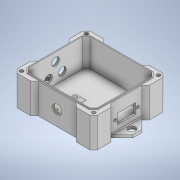
# Autodesk Inventor part: Case
Saved by Autodesk Inventor 2020 (Build 240168000, 168)
## iProperties
Created: 2020-03-10
Part Number: Case
Material: Generic
Document SubType Name: Modeling
Designer: Alex
Density: 1 g/cm^3
Appearance: Default
Author: Alex
Autodesk Inventor part; units mm, degrees
ref_plane "YZ Plane" through (0, 0, 0) normal (1, 0, 0) x (0, 1, 0)
ref_plane "XZ Plane" through (0, 0, 0) normal (0, 1, 0) x (-1, 0, 0)
ref_plane "XY Plane" through (0, 0, 0) normal (0, 0, 1) x (1, 0, 0)
sketch "Sketch1" plane through (0, 0, 0) normal (0, 1, 0) x (-1, 0, 0)
  line L0 (40, -36) -> (-40, -36) construction
  line L1 (-40, -36) -> (-40, 36) construction
  line L2 (-40, 36) -> (40, 36) construction
  line L3 (40, 36) -> (40, -36) construction
  line L4 (21, -36) -> (25, -40)
  line L5 (25, -40) -> (40, -40)
  line L6 (40, -40) -> (44, -36)
  line L7 (44, -36) -> (44, -21)
  line L8 (44, -21) -> (40, -17)
  line L9 (40, 17) -> (44, 21)
  line L10 (44, 21) -> (44, 36)
  line L11 (44, 36) -> (40, 40)
  line L12 (40, 40) -> (25, 40)
  line L13 (25, 40) -> (21, 36)
  line L14 (40, -17) -> (40, 17)
  line L15 (21, -36) -> (-21, -36)
  line L16 (-21, -36) -> (-25, -40)
  line L17 (-25, -40) -> (-40, -40)
  line L18 (-40, -40) -> (-44, -36)
  line L19 (-44, -36) -> (-44, -21)
  line L20 (-44, -21) -> (-40, -17)
  line L21 (-40, -17) -> (-40, 17)
  line L22 (-40, 17) -> (-44, 21)
  line L23 (-44, 21) -> (-44, 36)
  line L24 (-44, 36) -> (-40, 40)
  line L25 (-40, 40) -> (-25, 40)
  line L26 (-25, 40) -> (-21, 36)
  line L27 (21, 36) -> (-21, 36)
  line L28 (40, -36) -> (-40, 36) construction
  line L29 (-40, -36) -> (40, 36) construction
  point P0 (0, 0)
  point P1 (40, 0)
  point P2 (0, -36)
  point P3 (0, 0)
  point P4 (0, 36)
  point P5 (-40, 0)
  dimension "d0" = 4
  dimension "d1" = 80
  dimension "d2" = 72
  dimension "d3" = 4
  dimension "d4" = 4
  dimension "d5" = 4
  dimension "d6" = 135
  dimension "d7" = 0
  dimension "d8" = 15
  constraints: 60 end point, 13 parallel, 10 point on line, 7 equal length, 7 midpoint, 7 perpendicular, 6 collinear, 2 horizontal, 1 coincident, 1 horizontal alignment, 1 vertical alignment
  measures "d0" distance between parallel lines of L5 L0
  measures "d1" distance between parallel lines of L1 L3
  measures "d2" distance of L2.end L0.start
  measures "d3" distance between parallel lines of L7 L3
  measures "d4" distance between parallel lines of L19 L1
  measures "d5" distance between parallel lines of L25 L2
  measures "d6" angle of L15 L16
  measures "d7" distance from line of L17.end L1
  measures "d8" distance of L16.end L17.end
extrude "Extrusion1" add sketch "Sketch1" along normal blind 3
sketch "Sketch2" plane through (0, 3, 0) normal (0, 1, 0) x (1, 0, 0)
  line L0 (21, 36) -> (-21, 36) projected
  line L1 (-21, 36) -> (-25, 40) projected
  line L2 (-25, 40) -> (-40, 40) projected
  line L3 (-40, 40) -> (-44, 36) projected
  line L4 (-44, 36) -> (-44, 21) projected
  line L5 (-44, 21) -> (-40, 17) projected
  line L6 (-40, 17) -> (-40, -17) projected
  line L7 (-40, -17) -> (-44, -21) projected
  line L8 (-44, -21) -> (-44, -36) projected
  line L9 (-44, -36) -> (-40, -40) projected
  line L10 (-40, -40) -> (-25, -40) projected
  line L11 (-25, -40) -> (-21, -36) projected
  line L12 (-21, -36) -> (21, -36) projected
  line L13 (21, -36) -> (25, -40) projected
  line L14 (25, -40) -> (40, -40) projected
  line L15 (40, -40) -> (44, -36) projected
  line L16 (44, -36) -> (44, -21) projected
  line L17 (44, -21) -> (40, -17) projected
  line L18 (40, -17) -> (40, 17) projected
  line L19 (40, 17) -> (44, 21) projected
  line L20 (44, 21) -> (44, 36) projected
  line L21 (44, 36) -> (40, 40) projected
  line L22 (40, 40) -> (25, 40) projected
  line L23 (25, 40) -> (21, 36) projected
  line L24 (-21.8284, 34) -> (21.8284, 34)
  line L25 (21.8284, 34) -> (25.8284, 38) construction
  line L26 (25.8284, 38) -> (39.1716, 38) construction
  line L27 (39.1716, 38) -> (42, 35.1716) construction
  line L28 (42, 35.1716) -> (42, 21.8284) construction
  line L29 (42, 21.8284) -> (38, 17.8284) construction
  line L30 (38, 17.8284) -> (38, -17.8284)
  line L31 (38, -17.8284) -> (42, -21.8284) construction
  line L32 (42, -21.8284) -> (42, -35.1716) construction
  line L33 (42, -35.1716) -> (39.1716, -38) construction
  line L34 (39.1716, -38) -> (25.8284, -38) construction
  line L35 (25.8284, -38) -> (21.8284, -34) construction
  line L36 (21.8284, -34) -> (-21.8284, -34)
  line L37 (-21.8284, -34) -> (-25.8284, -38) construction
  line L38 (-25.8284, -38) -> (-39.1716, -38) construction
  line L39 (-39.1716, -38) -> (-42, -35.1716) construction
  line L40 (-42, -35.1716) -> (-42, -21.8284) construction
  line L41 (-42, -21.8284) -> (-38, -17.8284) construction
  line L42 (-38, -17.8284) -> (-38, 17.8284)
  line L43 (-38, 17.8284) -> (-42, 21.8284) construction
  line L44 (-42, 21.8284) -> (-42, 35.1716) construction
  line L45 (-42, 35.1716) -> (-39.1716, 38) construction
  line L46 (-39.1716, 38) -> (-25.8284, 38) construction
  line L47 (-25.8284, 38) -> (-21.8284, 34) construction
  line L48 (-38, 17.8284) -> (-38, 30)
  line L49 (-38, 30) -> (-34, 34)
  line L50 (-34, 34) -> (-21.8284, 34)
  line L51 (21.8284, 34) -> (34, 34)
  line L52 (34, 34) -> (38, 30)
  line L53 (38, 30) -> (38, 17.8284)
  line L54 (38, -17.8284) -> (38, -30)
  line L55 (38, -30) -> (34, -34)
  line L56 (34, -34) -> (21.8284, -34)
  line L57 (-21.8284, -34) -> (-34, -34)
  line L58 (-34, -34) -> (-38, -30)
  line L59 (-38, -30) -> (-38, -17.8284)
  point P0 (0, 0)
  dimension "d11" = 2
  dimension "d13" = 4
  constraints: 72 end point, 3 equal length, 3 perpendicular, 3 vertical, 2 parallel, 2 point on line, 1 collinear, 1 horizontal, 23 other
  measures "d11" distance between parallel lines of L0 L24
  measures "d13" horizontal distance of L49.end L48.end
extrude "Extrusion2" add sketch "Sketch2" along normal blind 30
sketch "Sketch3" plane through (0, 3, 0) normal (0, 1, 0) x (1, 0, 0)
  line L0 (-34, 34) -> (-38, 30) construction
  line L1 (-38, 30) -> (-38, -30) construction
  line L2 (-38, -30) -> (-34, -34) construction
  line L3 (-34, -34) -> (34, -34) construction
  line L4 (34, -34) -> (38, -30) construction
  line L5 (38, -30) -> (38, 30) construction
  line L6 (38, 30) -> (34, 34) construction
  line L7 (34, 34) -> (-34, 34) construction
  line L8 (21, -36) -> (25, -40) construction
  line L9 (25, -40) -> (40, -40) construction
  line L10 (40, -40) -> (44, -36) construction
  line L11 (44, -36) -> (44, -21) construction
  line L12 (44, -21) -> (40, -17) construction
  line L13 (40, -17) -> (40, 17) construction
  line L14 (40, 17) -> (44, 21) construction
  line L15 (44, 21) -> (44, 36) construction
  line L16 (44, 36) -> (40, 40) construction
  line L17 (40, 40) -> (25, 40) construction
  line L18 (25, 40) -> (21, 36) construction
  line L19 (21, 36) -> (-21, 36) construction
  line L20 (-21, 36) -> (-25, 40) construction
  line L21 (-25, 40) -> (-40, 40) construction
  line L22 (-40, 40) -> (-44, 36) construction
  line L23 (-44, 36) -> (-44, 21) construction
  line L24 (-44, 21) -> (-40, 17) construction
  line L25 (-40, 17) -> (-40, -17) construction
  line L26 (-40, -17) -> (-44, -21) construction
  line L27 (-44, -21) -> (-44, -36) construction
  line L28 (-44, -36) -> (-40, -40) construction
  line L29 (-40, -40) -> (-25, -40) construction
  line L30 (-25, -40) -> (-21, -36) construction
  line L31 (-21, -36) -> (21, -36) construction
  line L32 (-34, 34) -> (34, 34) construction
  line L33 (34, 34) -> (38, 30) construction
  line L34 (38, 30) -> (38, -30) construction
  line L35 (38, -30) -> (34, -34) construction
  line L36 (34, -34) -> (-34, -34) construction
  line L37 (-34, -34) -> (-38, -30) construction
  line L38 (-38, -30) -> (-38, 30) construction
  line L39 (-38, 30) -> (-34, 34) construction
  line L40 (-17.5, 32) -> (28, 32) construction
  line L41 (28, 32) -> (28, -10) construction
  line L42 (28, -10) -> (-17.5, -10) construction
  line L43 (-17.5, -10) -> (-17.5, 32) construction
  line L44 (-15.3, -0.9) -> (-9.3, -0.9)
  line L45 (-9.3, -0.9) -> (-9.3, -6.9)
  line L46 (-9.3, -6.9) -> (-15.3, -6.9)
  line L47 (-15.3, -6.9) -> (-15.3, -0.9)
  line L48 (20.4, 30.9) -> (26.4, 30.9)
  line L49 (26.4, 30.9) -> (26.4, 24.9)
  line L50 (26.4, 24.9) -> (20.4, 24.9)
  line L51 (20.4, 24.9) -> (20.4, 30.9)
  line L52 (-15.3, -0.9) -> (-9.3, -6.9) construction
  line L53 (-9.3, -0.9) -> (-15.3, -6.9) construction
  line L54 (20.4, 30.9) -> (26.4, 24.9) construction
  line L55 (26.4, 30.9) -> (20.4, 24.9) construction
  point P0 (0, 0)
  point P1 (-12.3, -3.9)
  point P2 (23.4, 27.9)
  dimension "d16" = 45.5
  dimension "d17" = 42
  dimension "d18" = 6
  dimension "d19" = 5.2
  dimension "d20" = 6.1
  dimension "d21" = 4.6
  dimension "d22" = 4.1
  dimension "d25" = 2
  dimension "d26" = 10
  constraints: 32 end point, 6 parallel, 5 perpendicular, 3 equal length, 3 horizontal, 2 midpoint
  measures "d16" distance of L40.start L40.end
  measures "d17" distance of L42.end L40.start
  measures "d18" distance of L44.end L45.end
  measures "d19" distance from line of L43 point (-12.3, -3.9)
  measures "d20" distance from line of point (-12.3, -3.9) L42
  measures "d21" distance from line of point (23.4, 27.9) L41
  measures "d22" distance from line of L40 point (23.4, 27.9)
  measures "d25" distance between parallel lines of L7 L40
  measures "d26" distance between parallel lines of L5 L41
extrude "Extrusion3" add sketch "Sketch3" along normal blind 3
chamfer "Chamfer1" distance 3 angle 45 8 edges at (-12.3, 3, 6.9) (-9.3, 3, 3.9) (-12.3, 3, 0.9) (-15.3, 3, 3.9) (20.4, 3, -27.9) (23.4, 3, -24.9) (26.4, 3, -27.9) (23.4, 3, -30.9)
sketch "Sketch4" plane through (0, 6, 0) normal (0, 1, 0) x (1, 0, 0)
  line L0 (-15.3, -6.9) -> (-9.3, -6.9) construction
  line L1 (-9.3, -6.9) -> (-9.3, -0.9) construction
  line L2 (-9.3, -0.9) -> (-15.3, -0.9) construction
  line L3 (-15.3, -0.9) -> (-15.3, -6.9) construction
  line L4 (26.4, 24.9) -> (26.4, 30.9) construction
  line L5 (26.4, 30.9) -> (20.4, 30.9) construction
  line L6 (20.4, 30.9) -> (20.4, 24.9) construction
  line L7 (20.4, 24.9) -> (26.4, 24.9) construction
  point P0 (0, 0)
  point P1 (-12.3, -3.9)
  point P2 (23.4, 27.9)
  point P3 (-15.3, -3.9)
  point P4 (20.4, 27.9)
  point P5 (23.4, 30.9)
  point P6 (-12.3, -0.9)
  constraints: 4 midpoint, 2 horizontal alignment, 2 vertical alignment
hole "Hole1" at (-12.3, 6, 3.9) at (23.4, 6, -27.9) direction (0, -1, 0) diameter 4 depth 5
hole "Hole2" at (0, 16.5, 36) direction (0, 0, -1) diameter 10 depth 2
sketch "Sketch6" plane through (40, 0, 17) normal (1, 0, 0) x (0, 0, -1)
  line L0 (1.5, 21) -> (32.5, 21) construction
  line L1 (32.5, 21) -> (32.5, 8) construction
  line L2 (32.5, 8) -> (1.5, 8) construction
  line L3 (1.5, 8) -> (1.5, 21) construction
  line L4 (7, 20) -> (27, 20)
  line L5 (27, 20) -> (27, 9)
  line L6 (27, 9) -> (7, 9)
  line L7 (7, 9) -> (7, 20)
  line L8 (0, 0) -> (34, 0) construction
  line L9 (34, 0) -> (34, 33) construction
  line L10 (0, 33) -> (34, 33) construction
  line L11 (0, 0) -> (0, 33) construction
  circle A0 centre (4.5, 14.5) radius 1.55
  circle A1 centre (29.5, 14.5) radius 1.55
  line L12 (4.5, 14.5) -> (29.5, 14.5) construction
  point P0 (17, 0)
  point P1 (32.5, 14.5)
  point P2 (27, 14.5)
  point P3 (17, 21)
  point P4 (17, 20)
  point P5 (17, 8)
  point P6 (17, 0)
  point P7 (1.5, 14.5)
  point P8 (17, 14.5)
  dimension "d48" = 31
  dimension "d49" = 13
  dimension "d50" = 20
  dimension "d51" = 11
  dimension "d52" = 8
  dimension "d53" = 25
  dimension "d54" = 3.1
  constraints: 18 end point, 8 midpoint, 4 parallel, 3 horizontal, 3 horizontal alignment, 3 vertical alignment, 2 centre point, 2 perpendicular, 1 equal radius
  measures "d48" distance of L0.start L0.end
  measures "d49" distance of L0.end L1.end
  measures "d50" distance of L4.start L4.end
  measures "d51" distance of L4.end L5.end
  measures "d52" distance between parallel lines of L2 L8
  measures "d53" distance of L12.end L12.start
  measures "d54" diameter of A0
extrude "Extrusion4" cut sketch "Sketch6" against normal blind 3
sketch "Sketch7" plane through (-40, 0, -17) normal (-1, 0, 0) x (0, 0, 1)
  circle A0 centre (17, 24.9904) radius 4.25
  circle A1 centre (9.5, 12) radius 4.25
  circle A2 centre (24.5, 12) radius 4.25
  line L0 (9.5, 12) -> (17, 24.9904) construction
  line L1 (17, 24.9904) -> (24.5, 12) construction
  line L2 (24.5, 12) -> (9.5, 12) construction
  line L3 (13.25, 18.4952) -> (24.5, 12) construction
  line L4 (9.5, 12) -> (20.75, 18.4952) construction
  line L5 (17, 24.9904) -> (17, 12) construction
  line L6 (0, 0) -> (34, 0) construction
  line L7 (34, 0) -> (34, 33) construction
  line L8 (0, 33) -> (34, 33) construction
  line L9 (0, 0) -> (0, 33) construction
  point P0 (17, 0)
  point P1 (17, 16.3301)
  point P2 (34, 16.5)
  point P3 (17, 33)
  dimension "d57" = 8.5
  dimension "d58" = 15
  dimension "d61" = 12
  constraints: 12 end point, 5 midpoint, 3 centre point, 2 equal length, 2 equal radius, 2 point on line, 1 horizontal, 1 vertical alignment
  measures "d57" diameter of A1
  measures "d58" distance of L1.end L0.start
  measures "d61" distance between parallel lines of L6 L2
extrude "Extrusion5" cut sketch "Sketch7" against normal blind 3
lip "Lip1" kind lip height 1 width 1 edges at (36, 33, -32) (0, 33, -34) (38, 33, 0) (36, 33, 32) (0, 33, 34) (-36, 33, 32) (-38, 33, 0) (-36, 33, -32) guide face at (7, 33, -34.6667)
sketch "Sketch8" plane through (0, 33, 0) normal (0, 1, 0) x (1, 0, 0)
  line L0 (-34.4142, 35) -> (34.4142, 35) construction
  line L1 (34.4142, 35) -> (39, 30.4142) construction
  line L2 (39, 30.4142) -> (39, -30.4142) construction
  line L3 (39, -30.4142) -> (34.4142, -35) construction
  line L4 (34.4142, -35) -> (-34.4142, -35) construction
  line L5 (-34.4142, -35) -> (-39, -30.4142) construction
  line L6 (-39, -30.4142) -> (-39, 30.4142) construction
  line L7 (-39, 30.4142) -> (-34.4142, 35) construction
  line L8 (44, 21) -> (44, 36) construction
  line L9 (44, 36) -> (40, 40) construction
  line L10 (40, 40) -> (25, 40) construction
  line L11 (25, 40) -> (21, 36) construction
  line L12 (21, 36) -> (-21, 36) construction
  line L13 (-21, 36) -> (-25, 40) construction
  line L14 (-25, 40) -> (-40, 40) construction
  line L15 (-40, 40) -> (-44, 36) construction
  line L16 (-44, 36) -> (-44, 21) construction
  line L17 (-44, 21) -> (-40, 17) construction
  line L18 (-40, 17) -> (-40, -17) construction
  line L19 (-40, -17) -> (-44, -21) construction
  line L20 (-44, -21) -> (-44, -36) construction
  line L21 (-44, -36) -> (-40, -40) construction
  line L22 (-40, -40) -> (-25, -40) construction
  line L23 (-25, -40) -> (-21, -36) construction
  line L24 (-21, -36) -> (21, -36) construction
  line L25 (21, -36) -> (25, -40) construction
  line L26 (25, -40) -> (40, -40) construction
  line L27 (40, -40) -> (44, -36) construction
  line L28 (44, -36) -> (44, -21) construction
  line L29 (44, -21) -> (40, -17) construction
  line L30 (40, -17) -> (40, 17) construction
  line L31 (40, 17) -> (44, 21) construction
  line L32 (-39.5341, -35.5341) -> (39.5341, 35.5341) construction
  line L33 (-39.5341, 35.5341) -> (39.5341, -35.5341) construction
  line L34 (40, 40) -> (39, 30.4142) construction
  line L35 (44, 36) -> (40, 40) construction
  line L36 (39, 30.4142) -> (34.4142, 35) construction
  line L37 (44, 36) -> (34.4142, 35) construction
  point P0 (0, 0)
  point P1 (0, 0)
  constraints: 8 end point, 2 horizontal alignment, 2 point on line, 2 vertical alignment, 1 coincident, 1 midpoint
hole "Hole3" at (39.5341, 33, -35.5341) at (39.5341, 33, 35.5341) at (-39.5341, 33, 35.5341) at (-39.5341, 33, -35.5341) direction (0, -1, 0) diameter 4 depth 5
sketch "Sketch9" plane through (0, 0, 0) normal (0, -1, 0) x (1, 0, 0)
  line L0 (-44, 21) -> (-44, 36) construction
  line L1 (-40, 17) -> (-44, 21) construction
  line L2 (-40, -17) -> (-40, 17) construction
  line L3 (-44, -21) -> (-40, -17) construction
  line L4 (-44, -36) -> (-44, -21) construction
  line L5 (-40, -40) -> (-44, -36) construction
  line L6 (-25, -40) -> (-40, -40) construction
  line L7 (-21, -36) -> (-25, -40) construction
  line L8 (21, -36) -> (-21, -36) construction
  line L9 (25, -40) -> (21, -36) construction
  line L10 (40, -40) -> (25, -40) construction
  line L11 (44, -36) -> (40, -40) construction
  line L12 (44, -21) -> (44, -36) construction
  line L13 (40, -17) -> (44, -21) construction
  line L14 (40, 17) -> (40, -17) construction
  line L15 (44, 21) -> (40, 17) construction
  line L16 (44, 36) -> (44, 21) construction
  line L17 (40, 40) -> (44, 36) construction
  line L18 (25, 40) -> (40, 40) construction
  line L19 (21, 36) -> (25, 40) construction
  line L20 (-21, 36) -> (21, 36) construction
  line L21 (-25, 40) -> (-21, 36) construction
  line L22 (-40, 40) -> (-25, 40) construction
  line L23 (-44, 36) -> (-40, 40) construction
  line L24 (40, -17) -> (52, -5)
  line L25 (52, -5) -> (52, 5)
  line L26 (52, 5) -> (40, 17)
  line L27 (40, -17) -> (40, 17)
  line L28 (0, -36) -> (0, 36) construction
  line L29 (-21, 36) -> (21, 36) construction
  circle A0 centre (46, 0) radius 4
  line L30 (52, 0) -> (40, 0) construction
  line L31 (40, 17) -> (40, -17) construction
  line L32 (-40, -17) -> (-44, -21) construction
  line L33 (-40, 17) -> (-40, -17) construction
  line L34 (-44, 21) -> (-40, 17) construction
  line L35 (-40, -17) -> (-52, -5)
  line L36 (-52, -5) -> (-52, 5)
  line L37 (-52, 5) -> (-40, 17)
  line L38 (-40, -17) -> (-40, 17)
  circle A1 centre (-46, 0) radius 4
  line L39 (-52, 0) -> (-40, 0) construction
  line L40 (-40, 17) -> (-40, -17) construction
  point P0 (0, 0)
  point P1 (46, 0)
  point P2 (-46, 0)
  dimension "d75" = 135
  dimension "d76" = 12
  dimension "d77" = 8
  constraints: 30 end point, 6 symmetric about line, 5 midpoint, 2 centre point, 2 coincident, 1 perpendicular, 1 vertical, 1 other
  measures "d75" angle of L14 L24
  measures "d76" distance between parallel lines of L14 L25
  measures "d77" diameter of A0
extrude "Extrusion6" add sketch "Sketch9" against normal blind 3
chamfer "Chamfer2" distance 1 angle 45 2 edges at (40, 3, 0) (-40, 3, 0)
equation "\"d3\" = d0"
equation "\"d4\" = d0"
equation "\"d5\" = d0"
body "Solid1"
